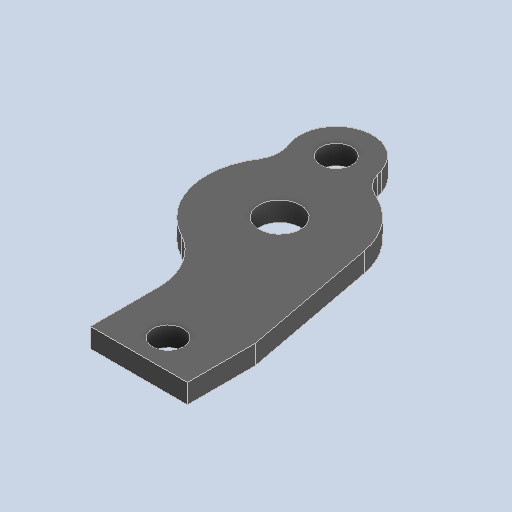
# Autodesk Inventor part: screw_lift_upper
Saved by Autodesk Inventor 2024.1 (Build 281209000, 209)
## iProperties
Created: 2025-01-18
Part Number: screw_lift_upper
Material: 一般
Document SubType Name: Modeling
Designer: hibik
Density: 1 g/cm^3
Appearance: 既定
Author: hibik
Autodesk Inventor part; units mm, degrees
ref_plane "YZ Plane" through (0, 0, 0) normal (1, 0, 0) x (0, 1, 0)
ref_plane "XZ Plane" through (0, 0, 0) normal (0, 1, 0) x (-1, 0, 0)
ref_plane "XY Plane" through (0, 0, 0) normal (0, 0, 1) x (1, 0, 0)
sketch "スケッチ1" plane through (0, 0, 0) normal (0, 1, 0) x (-1, 0, 0)
  line L0 (0, 0) -> (-19.1969, -33.25)
  line L1 (-19.1969, -33.25) -> (-10.9697, -38)
  line L2 (-10.9697, -38) -> (10.656, -38)
  line L3 (23.0438, 0) -> (-50.7627, 0) projected
  circle A0 centre (0, -50.5) radius 12.5
  line L4 (-19.1969, -33.25) -> (-30, -51.9615)
  line L5 (-30, -51.9615) -> (-40.219, -46.0616) construction
  line L6 (-30, -51.9615) -> (-24.5152, -61.4615)
  line L7 (-10.9697, -38) -> (-24.5152, -61.4615)
  line L8 (-24.5152, -61.4615) -> (-14.7652, -44.574)
  line L9 (-14.7652, -44.574) -> (-9.2226, -47.774)
  line L10 (-9.2226, -47.774) -> (-18.9726, -64.6615)
  line L11 (-18.9726, -64.6615) -> (-24.5152, -61.4615)
  line L12 (-10, -38) -> (-10, -31)
  line L13 (-10, -31) -> (0, -31)
  line L14 (0, -31) -> (0, -38)
  line L15 (2.0207, -47) -> (4.0415, -50.5)
  line L16 (4.0415, -50.5) -> (2.0207, -54)
  line L17 (2.0207, -54) -> (-2.0207, -54)
  line L18 (-2.0207, -54) -> (-4.0415, -50.5)
  line L19 (-4.0415, -50.5) -> (-2.0207, -47)
  line L20 (-2.0207, -47) -> (2.0207, -47)
  circle A1 centre (0, -50.5) radius 7.5
  arc A2 (0, -38) -> (3.5294, -43.8824) centre (6.6667, -38) ccw
  line L21 (-10, -38) -> (-7.3691, -51.8953)
  line L22 (-14.2226, -56.4343) -> (-18.5527, -53.9343)
  line L23 (-18.5527, -53.9343) -> (-13.5527, -45.274)
  line L24 (-13.5527, -45.274) -> (-9.2226, -47.774)
  line L25 (-9.2226, -47.774) -> (-14.2226, -56.4343)
  line L26 (-13.5527, -45.274) -> (-9.2294, -42.0698)
  line L27 (-14.2226, -56.4343) -> (-0.8456, -57.9522)
  circle A3 centre (0, -50.5) radius 2.15
  dimension "d0" = 38
  dimension "d1" = 60
  dimension "d2" = 9.5
  dimension "d3" = 25
  dimension "d4" = 60
  dimension "d5" = 60
  dimension "d6" = 19.5
  dimension "d7" = 6.4
  dimension "d8" = 10
  dimension "d9" = 7
  dimension "d10" = 7
  dimension "d11" = 15
  dimension "d12" = 5
  dimension "d13" = 10
  dimension "d19" = 4.3
  constraints: 54 end point, 7 point on circle, 5 parallel, 5 perpendicular, 5 point on line, 5 tangent, 4 centre point, 3 coincident, 3 horizontal, 2 collinear, 2 vertical, 1 vertical alignment, 13 other
  measures "d0" distance from line of L0.start L2
  measures "d1" angle of L3 L0
  measures "d2" distance from line of L1.end L0
  measures "d3" diameter of A0
  measures "d4" distance from line of L0.start L5
  measures "d5" angle of L4 L6
  measures "d6" distance between parallel lines of L11 L9
  measures "d7" distance between parallel lines of L7 L10
  measures "d8" distance of L12.end L13.end
  measures "d9" distance between parallel lines of L2 L13
  measures "d10" distance between parallel lines of L20 L17
  measures "d11" diameter of A1
  measures "d12" distance between parallel lines of L25 L23
  measures "d13" distance between parallel lines of L9 L22
  measures "d19" diameter of A3
extrude "押し出し1" add sketch "スケッチ1" along normal blind 2 contours L12 L13 L14 L2 | L2 A0 L21 | A2 A1 L21 A0 | A1 | L15 L16 L17 L18 L19 L20
sketch "スケッチ3" plane through (0, 2, 0) normal (0, 1, 0) x (1, 0, 0)
  circle A0 centre (5, 34) radius 1.6 projected
  circle A1 centre (-2.5376, 58.874) radius 1.6 projected
  line L0 (10, 31) -> (10, 38) projected
  line L1 (10, 38) -> (7.3691, 51.8953) projected
  arc A2 (7.3691, 51.8953) -> (2.9482, 57.3963) centre (0, 50.5) ccw projected
  arc A3 (1.2564, 59.2847) -> (2.9482, 57.3963) centre (4.1274, 60.1548) ccw projected
  line L2 (1.2564, 59.2847) -> (1.0513, 59.9615) projected
  arc A4 (1.0513, 59.9615) -> (-6.1264, 57.7864) centre (-2.5376, 58.874) ccw projected
  line L3 (-6.1264, 57.7864) -> (-5.9213, 57.1097) projected
  arc A5 (-6.2803, 54.5998) -> (-5.9213, 57.1097) centre (-8.7924, 56.2397) ccw projected
  arc A6 (-6.2803, 54.5998) -> (-3.5294, 43.8824) centre (0, 50.5) ccw projected
  arc A7 (0, 38) -> (-3.5294, 43.8824) centre (-6.6667, 38) ccw projected
  line L4 (0, 38) -> (0, 31) projected
  line L5 (0, 31) -> (10, 31) projected
  line L6 (-2.0496, 46.95) -> (-4.0992, 50.5) projected
  line L7 (-4.0992, 50.5) -> (-2.0496, 54.05) projected
  line L8 (-2.0496, 54.05) -> (2.0496, 54.05) projected
  line L9 (2.0496, 54.05) -> (4.0992, 50.5) projected
  line L10 (4.0992, 50.5) -> (2.0496, 46.95) projected
  line L11 (2.0496, 46.95) -> (-2.0496, 46.95) projected
  circle A8 centre (5, 34) radius 1.6 projected
  circle A9 centre (-2.5376, 58.874) radius 1.6 projected
  line L12 (10, 31) -> (10, 38) projected
  line L13 (10, 38) -> (7.3691, 51.8953) projected
  arc A10 (7.3691, 51.8953) -> (2.9482, 57.3963) centre (0, 50.5) ccw projected
  arc A11 (1.2564, 59.2847) -> (2.9482, 57.3963) centre (4.1274, 60.1548) ccw projected
  line L14 (1.2564, 59.2847) -> (1.0513, 59.9615) projected
  arc A12 (1.0513, 59.9615) -> (-6.1264, 57.7864) centre (-2.5376, 58.874) ccw projected
  line L15 (-6.1264, 57.7864) -> (-5.9213, 57.1097) projected
  arc A13 (-6.2803, 54.5998) -> (-5.9213, 57.1097) centre (-8.7924, 56.2397) ccw projected
  arc A14 (-6.2803, 54.5998) -> (-3.5294, 43.8824) centre (0, 50.5) ccw projected
  arc A15 (0, 38) -> (-3.5294, 43.8824) centre (-6.6667, 38) ccw projected
  line L16 (0, 38) -> (0, 31) projected
  line L17 (0, 31) -> (10, 31) projected
  line L18 (-2.0496, 46.95) -> (-4.0992, 50.5) projected
  line L19 (-4.0992, 50.5) -> (-2.0496, 54.05) projected
  line L20 (-2.0496, 54.05) -> (2.0496, 54.05) projected
  line L21 (2.0496, 54.05) -> (4.0992, 50.5) projected
  line L22 (4.0992, 50.5) -> (2.0496, 46.95) projected
  line L23 (2.0496, 46.95) -> (-2.0496, 46.95) projected
  arc A16 (7.3691, 51.8953) -> (-3.5294, 43.8824) centre (0, 50.5) ccw projected
  arc A17 (7.3691, 51.8953) -> (-3.5294, 43.8824) centre (0, 50.5) ccw projected
  point P0 (0, 0)
  point P1 (-6.2803, 54.5998)
extrude "押し出し3" add sketch "スケッチ3" against normal up to surface (2 mm away) contours A1 A16 A5 L3 A4 L2 A3
sketch "スケッチ4" plane through (0, 2, 0) normal (0, 1, 0) x (1, 0, 0)
  arc A0 (-1.2753, 57.8908) -> (-3.0418, 57.3555) centre (-2.5376, 58.874) ccw projected
  circle A1 centre (-2.5376, 58.874) radius 1.6
  circle A2 centre (5, 34) radius 1.6 projected
  point P0 (0, 0)
  point P1 (-3.0418, 57.3555)
  point P2 (-1.2753, 57.8908)
  constraints: 1 centre point, 1 coincident, 1 concentric
extrude "押し出し4" cut sketch "スケッチ4" against normal blind 10
